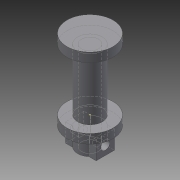
# Autodesk Inventor part: bearing v1
Saved by Autodesk Inventor 2015 (Build 190159000, 159)
## iProperties
Created: 2019-01-15
Part Number: bearing v1
Material: Generic
Document SubType Name: Modeling
Designer: Toby
Density: 1 g/cm^3
Appearance: Default
Author: Toby
Autodesk Inventor part; units mm, degrees
ref_plane "YZ Plane" through (0, 0, 0) normal (1, 0, 0) x (0, 1, 0)
ref_plane "XZ Plane" through (0, 0, 0) normal (0, 1, 0) x (-1, 0, 0)
ref_plane "XY Plane" through (0, 0, 0) normal (0, 0, 1) x (1, 0, 0)
sketch "Sketch1" plane through (0, 0, 0) normal (0, 0, 1) x (1, 0, 0)
  circle A0 centre (0, 0) radius 2.75
  circle A1 centre (0, 0) radius 4
  dimension "d0" = 5.5
  dimension "d1" = 8
  constraints: 2 centre point, 2 coincident
  measures "d0" diameter of A0
  measures "d1" diameter of A1
extrude "Extrusion1" add sketch "Sketch1" along normal blind 20
sketch "Sketch2" plane through (0, 0, 20) normal (0, 0, 1) x (1, 0, 0)
  circle A0 centre (0, 0) radius 7.5
  dimension "d4" = 15
  constraints: 1 centre point, 1 coincident
  measures "d4" diameter of A0
extrude "Extrusion2" add sketch "Sketch2" along normal blind 3
sketch "Sketch3" plane through (0, 0, 0) normal (1, 0, 0) x (0, 1, 0)
  point P0 (0, 0)
sketch "Sketch4" plane through (0, 0, 0) normal (0, 0, -1) x (-1, 0, 0)
  circle A0 centre (0, 0) radius 2.75
  circle A1 centre (0, 0) radius 7.5
  dimension "d7" = 5.5
  dimension "d8" = 15
  constraints: 2 centre point, 2 coincident
  measures "d7" diameter of A0
  measures "d8" diameter of A1
extrude "Extrusion3" add sketch "Sketch4" along normal blind 3
sketch "Sketch5" plane through (0, 0, -3) normal (0, 0, -1) x (-1, 0, 0)
  circle A0 centre (0, 0) radius 2.75
  circle A1 centre (0, 0) radius 4
  constraints: 2 centre point, 2 coincident
extrude "Extrusion4" add sketch "Sketch5" along normal blind 6
sketch "Sketch6" plane through (0, 0, 0) normal (1, 0, 0) x (0, 1, 0)
  circle A0 centre (0, -6) radius 1.5
  line L0 (-4, -9) -> (4, -9) projected
  point P0 (0, 0)
  dimension "d13" = 3
  dimension "d14" = 3
  constraints: 1 centre point
  measures "d13" diameter of A0
  measures "d14" distance from line of L0 A0.centre
extrude "Extrusion5" add sketch "Sketch6" along normal blind 6
sketch "Sketch7" plane through (6, 0, -6) normal (1, 0, 0) x (0, 0, -1)
  circle A0 centre (0, 0) radius 1.5 projected
  circle A1 centre (0, 0) radius 1.5
  point P0 (-6, 0)
  dimension "d17" = 3
  constraints: 1 centre point, 1 coincident
  measures "d17" diameter of A1
extrude "Extrusion6" cut sketch "Sketch7" against normal blind 20
sketch "Sketch8" plane through (0, 0, -3) normal (0, 0, -1) x (-1, 0, 0)
  line L0 (-5, 3) -> (-2.75, 3)
  line L1 (-2.75, 3) -> (-2.75, -3)
  line L2 (-2.75, -3) -> (-5, -3)
  line L3 (-5, -3) -> (-5, 3)
  line L4 (2.75, -3) -> (5, -3)
  line L5 (5, -3) -> (5, 3)
  line L6 (5, 3) -> (2.75, 3)
  line L7 (2.75, 3) -> (2.75, -3)
  point P0 (0, 0)
  dimension "d20" = 3
  dimension "d21" = 3
  dimension "d22" = 5
  dimension "d23" = 2.75
  dimension "d24" = 2.75
  dimension "d25" = 5
  constraints: 16 end point, 4 parallel, 2 horizontal, 2 perpendicular, 2 point on line
  measures "d20" distance from line of point (0, 0) L0
  measures "d21" distance from line of point (0, 0) L2
  measures "d22" distance from line of point (0, 0) L3
  measures "d23" distance from line of point (0, 0) L1
  measures "d24" distance from line of L7 point (0, 0)
  measures "d25" distance from line of point (0, 0) L5
extrude "Extrusion7" add sketch "Sketch8" along normal blind 6
sketch "Sketch9" plane through (5, -3, -3) normal (1, 0, 0) x (0, 0, -1)
  arc A0 (1.5, 3) -> (4.5, 3) centre (3, 3) ccw projected
  point P0 (-3, 3)
  constraints: 1 coincident
hole "Hole1" at (5, 0, -6) direction (-1, 0, 0) diameter 3 depth 8 tip angle 118
sketch "Sketch10" plane through (-5, -3, -3) normal (-1, 0, 0) x (0, 0, 1)
  circle A0 centre (-3, 3) radius 1.5 projected
  point P0 (3, 3)
  constraints: 1 coincident
hole "Hole2" at (-5, 0, -6) direction (1, 0, 0) diameter 3 depth 8 tip angle 118
body "Solid1"
